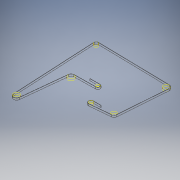
# Autodesk Inventor part: Belt 2
Saved by Autodesk Inventor 2016 (Build 200138000, 138)
## iProperties
Created: 2017-04-15
Part Number: Belt 2
Material: Rubber
Document SubType Name: Modeling
Designer: Scott
Density: 0.93 g/cm^3
Appearance: White
Author: Scott
Autodesk Inventor part; units mm, degrees
ref_plane "YZ Plane" through (0, 0, 0) normal (1, 0, 0) x (0, 1, 0)
ref_plane "XZ Plane" through (0, 0, 0) normal (0, 1, 0) x (-1, 0, 0)
sketch "Sketch1" plane through (0, 0, 0) normal (0, 0, 1) x (1, 0, 0)
  circle A0 centre (0, 0) radius 6.05
  constraints: 1 centre point, 1 coincident
surface extrude "ExtrusionSrf1" sketch "Sketch1" along normal mid plane 6 shown yes curves A0
sketch "Sketch2" plane through (0, 0, 0) normal (0, 0, 1) x (1, 0, 0)
  circle A0 centre (324.834, -10.3853) radius 6.05
  point P0 (0, 0)
  constraints: 1 centre point
surface extrude "ExtrusionSrf2" sketch "Sketch2" along normal mid plane 6 shown yes curves A0
sketch "Sketch3" plane through (0, 0, 0) normal (0, 0, 1) x (1, 0, 0)
  circle A0 centre (-9.3308, -291.8509) radius 6.11
  point P0 (0, 0)
  constraints: 1 centre point
surface extrude "ExtrusionSrf3" sketch "Sketch3" along normal blind 6 shown yes curves A0
sketch "Sketch4" plane through (0, 0, 0) normal (0, 0, 1) x (1, 0, 0)
  circle A0 centre (7.3217, -169.3662) radius 5.735
  point P0 (0, 0)
  constraints: 1 centre point
surface extrude "ExtrusionSrf4" sketch "Sketch4" along normal mid plane 6 shown yes curves A0
sketch "Sketch5" plane through (0, 0, 0) normal (0, 0, 1) x (1, 0, 0)
  circle A0 centre (319.839, -166.6212) radius 6.05
  point P0 (0, 0)
  constraints: 1 centre point
surface extrude "ExtrusionSrf5" sketch "Sketch5" along normal mid plane 6 shown yes curves A0
sketch "Sketch6" plane through (0, 0, 0) normal (0, 0, 1) x (1, 0, 0)
  circle A0 centre (160.3736, -162.9887) radius 3
  point P0 (0, 0)
  constraints: 1 centre point
surface extrude "ExtrusionSrf6" sketch "Sketch6" along normal mid plane 6 shown yes curves A0
sketch "Sketch7" plane through (0, 0, 0) normal (0, 0, 1) x (1, 0, 0)
  circle A0 centre (179.3639, -163.5958) radius 3
  point P0 (0, 0)
  constraints: 1 centre point
surface extrude "ExtrusionSrf7" sketch "Sketch7" along normal mid plane 6 shown yes curves A0
sketch "Sketch8" plane through (0, 0, 0) normal (0, 0, 1) x (1, 0, 0)
  circle A0 centre (0, 0) radius 6.05 projected
  circle A1 centre (7.3217, -169.3662) radius 5.735 projected
  circle A2 centre (-9.3308, -291.8509) radius 6.11 projected
  circle A3 centre (160.3736, -162.9887) radius 3 projected
  circle A4 centre (179.3639, -163.5958) radius 3 projected
  circle A5 centre (319.839, -166.6212) radius 6.05 projected
  circle A6 centre (324.834, -10.3853) radius 6.05 projected
  arc A7 (0.2015, 6.3018) -> (-6.3017, 0.2028) centre (0, 0) ccw
  arc A8 (-15.6925, -291.6462) -> (-2.969, -292.0543) centre (-9.3308, -291.8509) ccw
  arc A9 (7.4878, -163.0034) -> (0.9599, -169.1628) centre (7.3217, -169.3662) ccw
  arc A10 (160.2691, -166.9923) -> (160.4782, -158.985) centre (160.3736, -162.9887) ccw
  arc A11 (331.1358, -10.5868) -> (325.0355, -4.0835) centre (324.834, -10.3853) ccw
  arc A12 (179.5157, -159.5937) -> (179.2122, -167.5979) centre (179.3639, -163.5958) ccw
  arc A13 (319.6001, -172.9217) -> (326.1408, -166.8227) centre (319.839, -166.6212) ccw
  line L0 (-15.6925, -291.6462) -> (-6.3017, 0.2028)
  line L1 (0.2015, 6.3018) -> (325.0355, -4.0835)
  line L2 (-2.969, -292.0543) -> (0.9599, -169.1628)
  line L3 (7.4878, -163.0034) -> (160.2691, -166.9923)
  line L4 (331.1358, -10.5868) -> (326.1408, -166.8227)
  line L5 (148.4782, -158.6717) -> (160.4782, -158.985)
  line L6 (179.2122, -167.5979) -> (319.6001, -172.9217)
  line L7 (179.5157, -159.5937) -> (191.5157, -160.0488)
  dimension "d14" = 0.255
  dimension "d15" = 0.255
  dimension "d16" = 0.255
  dimension "d17" = 0.63
  dimension "d19" = 0.255
  dimension "d22" = 1.005
  dimension "d23" = 1.005
  dimension "d35" = 12
  dimension "d36" = 12
  constraints: 16 end point, 14 point on circle, 14 tangent, 7 centre point, 7 coincident, 2 parallel
  measures "d14" radial gap between concentric circles of A7 A0
  measures "d15" radial gap between concentric circles of A11 A6
  measures "d16" radial gap between concentric circles of A8 A2
  measures "d17" radial gap between concentric circles of A9 A1
  measures "d19" radial gap between concentric circles of A13 A5
  measures "d22" radial gap between concentric circles of A10 A3
  measures "d23" radial gap between concentric circles of A12 A4
  measures "d35" horizontal distance of L5.start L5.end
  measures "d36" horizontal distance of L7.start L7.end
ref_plane "Work Plane2" through (191.5157, -160.0488, 0) normal (0.9992817, -0.0378944, 0) x (0.0378944, 0.9992817, 0)
sketch "Sketch10" plane through (191.5157, -160.0488, 0) normal (0.9992817, -0.0378944, 0) x (0.0378944, 0.9992817, 0)
  line L0 (0.63, 3) -> (-0.255, 3)
  line L1 (-0.255, 3) -> (-0.255, -3)
  line L2 (-0.255, -3) -> (0.63, -3)
  line L3 (0.63, -3) -> (0.63, 3)
  line L4 (0.63, 0) -> (-0.255, 0) construction
  point P0 (152.6764, 0)
  point P1 (0, 0)
  dimension "d29" = 6
  dimension "d30" = 0.63
  dimension "d31" = 0.255
  constraints: 10 end point, 2 midpoint, 2 parallel, 1 horizontal, 1 perpendicular, 1 point on line
  measures "d29" distance of L2.end L0.start
  measures "d30" distance from line of point (0, 0) L3
  measures "d31" distance from line of L1 point (0, 0)
sweep "Sweep2" add profiles "Sketch10" path "Sketch8" path curves L7 A12 L6 A13 L4 A11 L1 A7 L0 A8 L2 A9 L3 A10 L5
equation "\"d14\" = inside"
equation "\"d15\" = inside"
equation "\"d16\" = inside"
equation "\"d17\" = backside"
equation "\"d19\" = inside"
equation "\"d30\" = backside"
equation "\"d31\" = inside"
equation "\"inside\" = 0.255"
equation "\"backside\" = 0.63"
body "Solid2"
body "Srf1"
body "Srf2"
body "Srf3"
body "Srf4"
body "Srf5"
body "Srf6"
body "Srf7"
